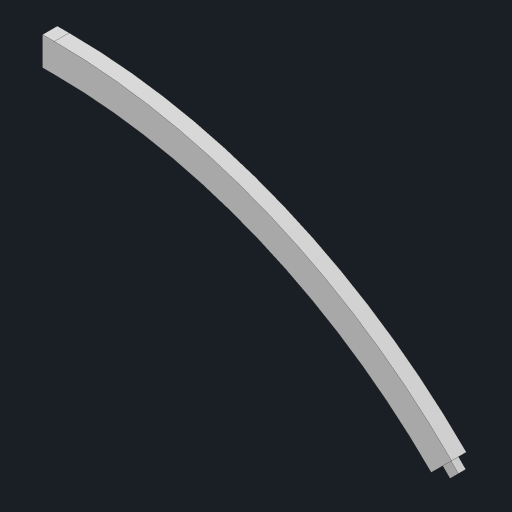
# Autodesk Inventor part: SEPARADOR_3
Saved by Autodesk Inventor 2024.3 (Build 283343000, 343)
## iProperties
Created: 2024-07-03
Part Number: SEPARADOR_3
Material: Generic
Document SubType Name: Modeling
Designer: Niler
Density: 1 g/cm^3
Appearance: Default
Author: Niler
Autodesk Inventor part; units mm, degrees
ref_plane "YZ Plane" through (0, 0, 0) normal (1, 0, 0) x (0, 1, 0)
ref_plane "XZ Plane" through (0, 0, 0) normal (0, 1, 0) x (-1, 0, 0)
ref_plane "XY Plane" through (0, 0, 0) normal (0, 0, 1) x (1, 0, 0)
sketch "Sketch1" plane through (0, 0, 0) normal (0, 0, 1) x (1, 0, 0)
  arc A0 (381.5, -381.5) -> (0, 0) centre (0, -381.5) ccw projected
  line L0 (-227, 0) -> (0, 0) projected
  line L1 (381.5, -381.5) -> (381.5, -681.5) projected
  line L2 (-227, -19.5) -> (0, -19.5)
  arc A1 (362, -381.5) -> (0, -19.5) centre (0, -381.5) ccw
  line L3 (362, -381.5) -> (362, -681.5)
  line L4 (-8, 0) -> (-8, -19.5)
  line L5 (381.5, -389.5) -> (362, -389.5)
  line L6 (269.7612, -111.7388) -> (255.9727, -125.5273)
  dimension "d0" = 19.5
  dimension "d1" = 8
  dimension "d2" = 8
  constraints: 10 end point, 4 point on circle, 4 point on line, 2 perpendicular, 1 centre point, 2 other
  measures "d0" radial gap between concentric circles of A0 A1
  measures "d1" distance from line of L5 L1.start
  measures "d2" distance from line of L4 L0.end
extrude "Extrusion1" add sketch "Sketch1" against normal blind 10 contours L6 A1 L2 L4 L0 A0
sketch "Sketch2" plane through (-8, -19.5, 0) normal (-1, 0, 0) x (0, 0, 1)
  line L0 (0, 19.5) -> (0, 0) projected
  line L1 (0, 19.5) -> (-10, 19.5) projected
  line L2 (-10, 0) -> (-10, 19.5) projected
  line L3 (0, 0) -> (-10, 0) projected
  line L4 (-1.2, 14.5) -> (-4.2, 14.5)
  line L5 (-4.2, 14.5) -> (-4.2, 9.5)
  line L6 (-4.2, 9.5) -> (-1.2, 9.5)
  line L7 (-1.2, 9.5) -> (-1.2, 14.5)
  line L8 (-1.2, 14.5) -> (-4.2, 9.5) construction
  line L9 (-4.2, 14.5) -> (-1.2, 9.5) construction
  point P0 (0, 19.5)
  point P1 (-2.7, 12)
  dimension "d5" = 3
  dimension "d6" = 5
  dimension "d7" = 1.2
  dimension "d8" = 5
  constraints: 12 end point, 2 midpoint, 2 parallel, 1 horizontal, 1 perpendicular
  measures "d5" distance of L6.end L5.end
  measures "d6" distance of L5.end L4.end
  measures "d7" distance between parallel lines of L0 L7
  measures "d8" distance between parallel lines of L1 L4
extrude "Extrusion2" cut sketch "Sketch2" against normal blind 7.1 contours L7 L6 L5 L4
sketch "Sketch3" plane through (255.9727, -125.5273, 0) normal (0.7071, -0.7071, 0) x (-0.7071, -0.7071, 0)
  line L0 (0, 0) -> (-19.5, 0) projected
  line L1 (0, 0) -> (0, 10) projected
  line L2 (-19.5, 10) -> (0, 10) projected
  line L3 (-19.5, 0) -> (-19.5, 10) projected
  line L4 (-15.5, 2.5) -> (-7.5, 2.5)
  line L5 (-7.5, 2.5) -> (-7.5, 7.5)
  line L6 (-7.5, 7.5) -> (-15.5, 7.5)
  line L7 (-15.5, 7.5) -> (-15.5, 2.5)
  line L8 (-15.5, 2.5) -> (-7.5, 7.5) construction
  line L9 (-7.5, 2.5) -> (-15.5, 7.5) construction
  point P0 (92.2388, 0)
  point P1 (-11.5, 5)
  point P2 (-15.5, 5)
  point P3 (-19.5, 5)
  dimension "d11" = 8
  dimension "d12" = 5
  dimension "d13" = 4
  constraints: 12 end point, 4 midpoint, 2 parallel, 1 horizontal, 1 horizontal alignment, 1 perpendicular
  measures "d11" distance of L6.end L5.end
  measures "d12" distance of L5.end L4.end
  measures "d13" distance between parallel lines of L7 L3
extrude "Extrusion3" add sketch "Sketch3" along normal blind 7 contours L7 L6 L5 L4
body "Solid1"
